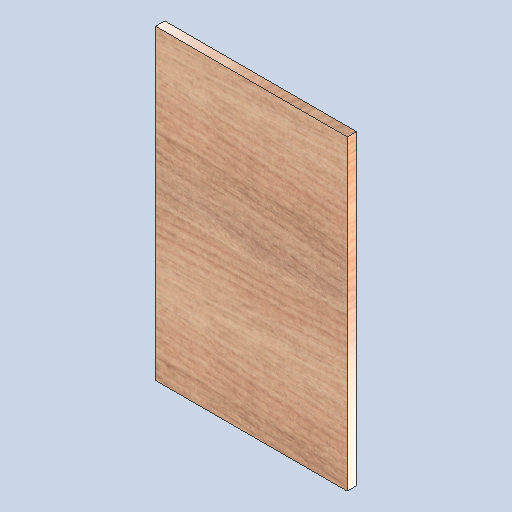
# Autodesk Inventor part: Deska_spodni
Saved by Autodesk Inventor 2024.2 (Build 282272000, 272)
## iProperties
Created: 2024-03-09
Part Number: Deska_spodni
Material: Dřevo (Bříza)
Document SubType Name: Modeling
Designer: lukyv
Density: 0.55 g/cm^3
Appearance: Bříza – přírodní leštěná
Author: lukyv
Autodesk Inventor part; units mm, degrees
ref_plane "YZ Plane" through (0, 0, 0) normal (1, 0, 0) x (0, 1, 0)
ref_plane "XZ Plane" through (0, 0, 0) normal (0, 1, 0) x (-1, 0, 0)
ref_plane "XY Plane" through (0, 0, 0) normal (0, 0, 1) x (1, 0, 0)
sketch "Náčrt1" plane through (0, 0, 0) normal (0, 1, 0) x (-1, 0, 0)
  line L0 (0, 0) -> (-250, 0)
  line L1 (-250, 0) -> (-250, -400)
  line L2 (-250, -400) -> (0, -400)
  line L3 (0, -400) -> (0, 0)
  dimension "d0" = 400
  dimension "d1" = 250
  constraints: 8 end point, 2 parallel, 1 horizontal, 1 perpendicular
  measures "d0" distance of L0.end L1.end
  measures "d1" distance of L1.end L2.end
extrude "Vysunutí1" add sketch "Náčrt1" along normal blind 12
